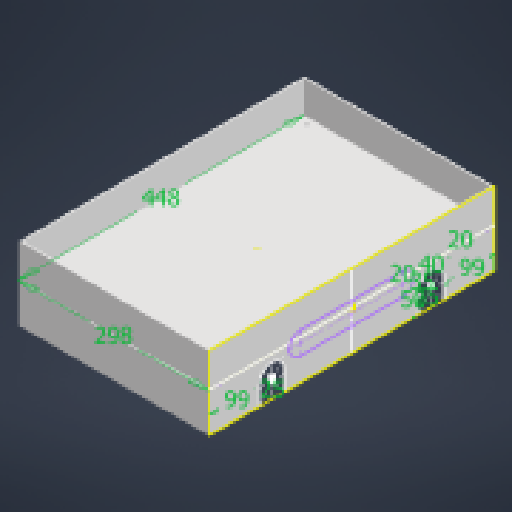
# Autodesk Inventor part: AMR_Top_Basket
Saved by Autodesk Inventor 2026.2 (Build 302298010, 298A)
## iProperties
Created: 2026-03-25
Part Number: AMR_Top_Basket
Material: Generic
Document SubType Name: Modeling
Designer: Srishanth Dhondy
Density: 1 g/cm^3
Appearance: Default
Author: Srishanth Dhondy
Autodesk Inventor part; units mm, degrees
ref_plane "YZ Plane" through (0, 0, 0) normal (1, 0, 0) x (0, 1, 0)
ref_plane "XZ Plane" through (0, 0, 0) normal (0, 1, 0) x (-1, 0, 0)
ref_plane "XY Plane" through (0, 0, 0) normal (0, 0, 1) x (1, 0, 0)
sketch "Sketch1" plane through (0, 0, 0) normal (0, 1, 0) x (-1, 0, 0)
  line L0 (-149, -224) -> (149, -224)
  line L1 (149, -224) -> (149, 224)
  line L2 (149, 224) -> (-149, 224)
  line L3 (-149, 224) -> (-149, -224)
  line L4 (-149, -224) -> (149, 224) construction
  line L5 (149, -224) -> (-149, 224) construction
  point P0 (0, 0)
  point P1 (132, 210)
  point P2 (-132, -210)
  point P3 (132, -210)
  point P4 (-132, 210)
  dimension "d0" = 298
  dimension "d1" = 448
  constraints: 12 end point, 2 midpoint, 2 parallel, 1 horizontal, 1 perpendicular
  measures "d0" distance of L2.end L1.end
  measures "d1" distance of L1.end L0.end
extrude "Extrusion1" add sketch "Sketch1" along normal blind 3
sketch "Sketch2" plane through (0, 3, 0) normal (0, 1, 0) x (1, 0, 0)
  line L0 (-149, 224) -> (-149, -224) projected
  line L1 (-149, -224) -> (149, -224) projected
  line L2 (149, -224) -> (149, 224) projected
  line L3 (149, 224) -> (-149, 224) projected
  line L4 (-149, 224) -> (-149, -224) projected
  line L5 (-149, -224) -> (149, -224) projected
  line L6 (149, -224) -> (149, 224) projected
  line L7 (149, 224) -> (-149, 224) projected
  line L8 (-146, -221) -> (-146, 221)
  line L9 (-146, 221) -> (146, 221)
  line L10 (146, 221) -> (146, -221)
  line L11 (146, -221) -> (-146, -221)
  point P0 (0, 0)
  dimension "d4" = 3
  constraints: 8 end point, 3 other
  measures "d4" distance between parallel lines of L0 L8
extrude "Extrusion2" add sketch "Sketch2" along normal blind 50 and the other way blind 65
hole "Hole1" at (132, 0, -210) at (132, 0, 210) at (-132, 0, 210) at (-132, 0, -210) direction (0, 1, 0) diameter 5 end through all
sketch "Sketch3" plane through (149, -62, -224) normal (1, 0, 0) x (0, 0, -1)
  line L0 (0, 0) -> (0, 115) projected
  line L1 (-448, 115) -> (0, 115) projected
  line L2 (-448, 0) -> (-448, 115) projected
  line L3 (0, 0) -> (-448, 0) projected
  point P0 (-224, 62)
sketch "Sketch4" plane through (149, -62, -224) normal (1, 0, 0) x (0, 0, -1)
  line L0 (0, 0) -> (0, 115) projected
  line L1 (-448, 115) -> (0, 115) projected
  line L2 (-448, 0) -> (-448, 115) projected
  line L3 (0, 0) -> (-448, 0) projected
  point P0 (-224, 62)
sketch "Sketch5" plane through (149, -62, -224) normal (1, 0, 0) x (0, 0, -1)
  line L0 (0, 0) -> (0, 115) projected
  line L1 (-448, 115) -> (0, 115) projected
  line L2 (-448, 0) -> (-448, 115) projected
  line L3 (0, 0) -> (-448, 0) projected
  line L4 (0, 0) -> (-448, 0) projected
  point P0 (-224, 62)
  point P1 (-224, 62)
  point P2 (-99, 25)
  dimension "d16" = 99
  dimension "d17" = 25
  measures "d16" horizontal distance of L0.start point (-99, 25)
  measures "d17" distance from line of L3 point (-99, 25)
sketch "Sketch6" plane through (149, -62, -224) normal (1, 0, 0) x (0, 0, -1)
  line L0 (0, 0) -> (-448, 0) projected
  line L1 (-445, 115) -> (-3, 115) projected
  line L2 (-224, 115) -> (-224, 0)
  line L3 (-79, 0) -> (-119, 0)
  line L4 (-119, 0) -> (-119, 30)
  line L5 (-99, 50) -> (-99, 50)
  line L6 (-79, 30) -> (-79, 0)
  line L7 (-79, 0) -> (-119, 50) construction
  line L8 (-119, 0) -> (-79, 50) construction
  line L9 (-448, 0) -> (-448, 115) projected
  arc A0 (-99, 50) -> (-119, 30) centre (-99, 30) ccw
  arc A1 (-79, 30) -> (-99, 50) centre (-99, 30) ccw
  line L10 (-329, 0) -> (-329, 30)
  line L11 (-369, 30) -> (-369, 0)
  line L12 (-369, 0) -> (-329, 50) construction
  line L13 (-329, 0) -> (-369, 50) construction
  arc A2 (-329, 30) -> (-349, 50) centre (-349, 30) ccw
  arc A3 (-349, 50) -> (-369, 30) centre (-349, 30) ccw
  line L14 (-304.3108, 54.0001) -> (-144.3108, 54.0001) construction
  line L15 (-445, 62) -> (-3, 62) projected
  line L16 (-304.3108, 36.5001) -> (-144.3108, 36.5001)
  line L17 (-144.3108, 71.5001) -> (-304.3108, 71.5001)
  arc A4 (-304.3108, 71.5001) -> (-304.3108, 36.5001) centre (-304.3108, 54.0001) ccw
  arc A5 (-144.3108, 36.5001) -> (-144.3108, 71.5001) centre (-144.3108, 54.0001) ccw
  point P0 (-224, 62)
  point P1 (-99, 25)
  point P2 (-99, 25)
  point P3 (-99, 25)
  point P4 (-119, 0)
  point P5 (-79, 0)
  point P6 (-349, 25)
  point P7 (-349, 25)
  point P8 (-99, 50)
  point P9 (-349, 50)
  point P10 (-329, 0)
  point P11 (-224.3108, 54.0001)
  point P12 (-304.3108, 54.0001)
  dimension "d18" = 40
  dimension "d19" = 50
  dimension "d26" = 20
  dimension "d27" = 20
  dimension "d28" = 99
  dimension "d29" = 25
  dimension "d32" = 35
  constraints: 30 end point, 12 point on circle, 11 symmetric about line, 8 tangent, 6 centre point, 6 midpoint, 6 point on line, 4 parallel, 2 coincident, 1 horizontal, 1 perpendicular, 2 other
  measures "d18" distance of L7.end L8.end
  measures "d19" distance of L3.end L7.end
  measures "d26" radius of A0
  measures "d27" radius of A1
  measures "d28" distance from line of L9 point (-349, 25)
  measures "d29" distance from line of point (-349, 25) L0
  measures "d32" diameter of A5
extrude "Extrusion3" cut sketch "Sketch6" against normal through all contours L0 L4 A0 A1 L6
extrude "Extrusion4" cut sketch "Sketch6" against normal through all contours L0 L11 A3 A2 L10
extrude "Extrusion5" cut sketch "Sketch6" against normal blind 3 contours L16 A4 L15 L2 | L2 L15 A5 L16 | L15 A4 L17 L2 | L2 L17 A5 L15
sketch "Sketch7" plane through (149, -62, -224) normal (1, 0, 0) x (0, 0, -1)
  arc A0 (-144.3108, 36.5001) -> (-144.3108, 71.5001) centre (-144.3108, 54.0001) ccw projected
  line L0 (-144.3108, 36.5001) -> (-304.3108, 36.5001) projected
  arc A1 (-304.3108, 71.5001) -> (-304.3108, 36.5001) centre (-304.3108, 54.0001) ccw projected
  line L1 (-304.3108, 71.5001) -> (-144.3108, 71.5001) projected
  line L2 (-369, 0) -> (-369, 30) projected
  arc A2 (-329, 30) -> (-369, 30) centre (-349, 30) ccw projected
  line L3 (-329, 30) -> (-329, 0) projected
  line L4 (-119, 0) -> (-329, 0) projected
  line L5 (-119, 0) -> (-119, 30) projected
  arc A3 (-79, 30) -> (-119, 30) centre (-99, 30) ccw projected
  line L6 (-79, 30) -> (-79, 0) projected
  line L7 (0, 0) -> (-79, 0) projected
  line L8 (0, 0) -> (0, 115) projected
  line L9 (-448, 115) -> (0, 115) projected
  line L10 (-448, 0) -> (-448, 115) projected
  line L11 (-369, 0) -> (-448, 0) projected
  point P0 (-224, 62)
ref_plane "Work Plane2" through (0, -62, -224) normal (1, 0, 0) x (0, 0, -1)
sketch "Sketch8" plane through (149, -62, -224) normal (1, 0, 0) x (0, 0, -1)
  arc A0 (-144.3108, 36.5001) -> (-144.3108, 71.5001) centre (-144.3108, 54.0001) ccw projected
  line L0 (-144.3108, 36.5001) -> (-304.3108, 36.5001) projected
  arc A1 (-304.3108, 71.5001) -> (-304.3108, 36.5001) centre (-304.3108, 54.0001) ccw projected
  line L1 (-304.3108, 71.5001) -> (-144.3108, 71.5001) projected
  line L2 (-369, 0) -> (-369, 30) projected
  arc A2 (-329, 30) -> (-369, 30) centre (-349, 30) ccw projected
  line L3 (-329, 30) -> (-329, 0) projected
  line L4 (-119, 0) -> (-329, 0) projected
  line L5 (-119, 0) -> (-119, 30) projected
  arc A3 (-79, 30) -> (-119, 30) centre (-99, 30) ccw projected
  line L6 (-79, 30) -> (-79, 0) projected
  line L7 (0, 0) -> (-79, 0) projected
  line L8 (0, 0) -> (0, 115) projected
  line L9 (-448, 115) -> (0, 115) projected
  line L10 (-448, 0) -> (-448, 115) projected
  line L11 (-369, 0) -> (-448, 0) projected
  point P0 (-224, 62)
mirror "Mirror1" about plane through (0, -62, -224) normal (1, 0, 0) of "Extrusion5"
body "Solid1"
